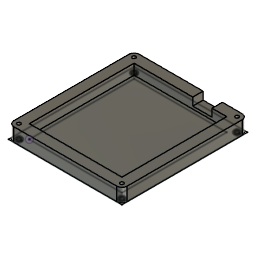
HackPad_bottom (Autodesk Fusion 360 design; units mm, degrees)
part number: 2025-12-18-10-40-01-433
Autodesk Fusion 360 part; units mm, degrees
sketch "Schizzo1" plane through (0, 0, 0) normal (0, 0, 1) x (1, 0, 0)
  line L0 (0, 0) -> (89.1, 0)
  line L1 (89.1, 0) -> (89.1, 100.8)
  line L2 (89.1, 100.8) -> (0, 100.8)
  line L3 (0, 100.8) -> (0, 0)
  line L4 (-10, -10) -> (99.1, -10)
  line L5 (99.1, -10) -> (99.1, 110.8)
  line L6 (99.1, 110.8) -> (-10, 110.8)
  line L7 (-10, 110.8) -> (-10, -10)
  circle A0 centre (94.1, 105.8) radius 1.7
  circle A1 centre (94.1, 105.8) radius 3
  circle A2 centre (94.1, -5) radius 1.7
  circle A3 centre (94.1, -5) radius 3
  circle A4 centre (-5, -5) radius 1.7
  circle A5 centre (-5, -5) radius 3
  circle A6 centre (-5, 105.8) radius 1.7
  circle A7 centre (-5, 105.8) radius 3
  dimension "d5" = 10
  dimension "d6" = 10
  dimension "d7" = 109.1
  dimension "d8" = 89.1
  dimension "d9" = 100.8
  dimension "d10" = 120.8
  dimension "d11" = 3.4
  dimension "d14" = 6
  dimension "d15" = 3.4
  dimension "d18" = 5
  dimension "d19" = 5
  dimension "d20" = 5
  dimension "d21" = 5
  dimension "d22" = 6
  dimension "d23" = 3.4
  dimension "d24" = 5
  dimension "d25" = 5
  dimension "d26" = 6
  dimension "d27" = 3.4
  dimension "d28" = 5
  dimension "d29" = 5
  dimension "d30" = 6
  constraint horizontal L0
  constraint vertical L1
  constraint horizontal L2
  constraint vertical L3
  constraint coincident L0.start L3.end
  constraint horizontal L4
  constraint vertical L5
  constraint horizontal L6
  constraint vertical L7
  constraint concentric A0 A1
  constraint concentric A2 A3
  constraint concentric A4 A5
  constraint concentric A6 A7
  measures "d5" distance of L2 L6
  measures "d6" distance of L1 L5
  measures "d7" distance of L5.end L6.end
  measures "d8" distance of L1.end L2.end
  measures "d9" distance of L0.end L1.end
  measures "d10" distance of L4.end L5.end
  measures "d11" diameter of A0
  measures "d14" diameter of A1
  measures "d15" diameter of A2
  measures "d18" distance of L4 A2.centre
  measures "d19" distance of L5 A2.centre
  measures "d20" distance of L5 A0.centre
  measures "d21" distance of L6 A0.centre
  measures "d22" diameter of A3
  measures "d23" diameter of A4
  measures "d24" distance of L4 A4.centre
  measures "d25" distance of L7 A4.centre
  measures "d26" diameter of A5
  measures "d27" diameter of A6
  measures "d28" distance of L6 A6.centre
  measures "d29" distance of L7 A6.centre
  measures "d30" diameter of A7
extrude "Estrusione1" add sketch "Schizzo1" along normal blind 9.9 from surface at 3.1 contours A1 | A3 | A5 | A7 makes body 1 at (94.9125, -2.1121, 9.7) makes body 2 at (-2.0037, -5.1495, 9.7) makes body 3 at (92.0053, 103.6524, 9.7) makes body 4 at (-2.1809, 104.7739, 9.7)
extrude "Estrusione2" add sketch "Schizzo1" along normal blind 13 contours L4 L5 L6 L7 bodies 1 2 3 4
extrude "Estrusione3" add sketch "Schizzo1" along normal blind 3 contours L0 L1 L2 L3 bodies 1
sketch "Schizzo2" plane through (0, 0, 13) normal (0, 0, 1) x (-1, 0, 0)
  circle A0 centre (-94.1, 5) radius 1.7
  circle A1 centre (5, -105.8) radius 1.7
  line L0 (0, 0) -> (0, -100.8)
  line L1 (0, -100.8) -> (-89.1, -100.8)
  line L2 (-89.1, -100.8) -> (-89.1, 0)
  line L3 (-89.1, 0) -> (0, 0)
  line L4 (10, -110.8) -> (10, 10)
  line L5 (10, 10) -> (-99.1, 10)
  line L6 (-99.1, 10) -> (-99.1, -110.8)
  line L7 (-99.1, -110.8) -> (10, -110.8)
  circle A2 centre (5, 5) radius 1.7
  circle A3 centre (-94.1, -105.8) radius 1.7
  line L8 (-56.455, -110.8) -> (-74.955, -110.8)
  line L9 (-74.955, -110.8) -> (-74.955, -100.8)
  line L10 (-74.955, -100.8) -> (-56.455, -100.8)
  line L11 (-56.455, -100.8) -> (-56.455, -110.8)
  line L12 (10, -110.8) -> (10, 10)
  dimension "d38" = 18.5
  dimension "d39" = 66.455
  constraint horizontal L8
  constraint vertical L9
  constraint horizontal L10
  constraint vertical L11
  constraint coincident L1 L9.end
  constraint coincident L7 L8.start
  measures "d38" distance of L8.start L8.end
  measures "d39" distance of L11 L12
extrude "Estrusione4" cut sketch "Schizzo2" against normal blind 7.5 contours L1 L7 L8 L9 L10 L11 bodies 1
fillet "Raccordo1" radius 5 4 edges at (99.1, -10, 6.5) (-10, -10, 6.5) (99.1, 110.8, 6.5) (-10, 110.8, 6.5) on bodies 1
